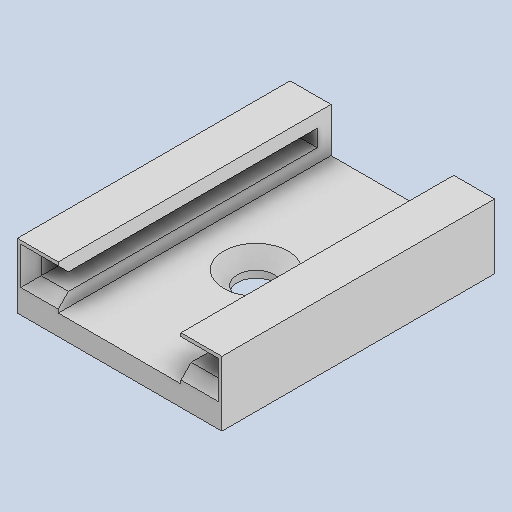
# Autodesk Inventor part: spodok_drazka
Saved by Autodesk Inventor 2025 (Build 290162000, 162)
## iProperties
Created: 2025-09-19
Part Number: spodok_drazka
Material: Generic
Document SubType Name: Modeling
Designer: Pravoslav
Density: 1 g/cm^3
Appearance: Default
Author: Pravoslav
Autodesk Inventor part; units mm, degrees
ref_plane "YZ Plane" through (0, 0, 0) normal (1, 0, 0) x (0, 1, 0)
ref_plane "XZ Plane" through (0, 0, 0) normal (0, 1, 0) x (-1, 0, 0)
ref_plane "XY Plane" through (0, 0, 0) normal (0, 0, 1) x (1, 0, 0)
sketch "Sketch1" plane through (0, 0, 0) normal (0, 1, 0) x (-1, 0, 0)
  line L0 (15, 20) -> (-15, 20)
  line L1 (-15, 20) -> (-15, -20)
  line L2 (-15, -20) -> (15, -20)
  line L3 (15, -20) -> (15, 20)
  line L4 (15, 20) -> (-15, -20) construction
  line L5 (-15, 20) -> (15, -20) construction
  circle A0 centre (0, 0) radius 2.75
  dimension "d0" = 30
  dimension "d1" = 40
  dimension "d2" = 5.5
  constraints: 12 end point, 2 midpoint, 2 parallel, 1 centre point, 1 coincident, 1 horizontal, 1 perpendicular
  measures "d0" distance of L2.end L1.end
  measures "d1" distance of L1.end L0.end
  measures "d2" diameter of A0
extrude "Extrusion1" add sketch "Sketch1" along normal blind 3
chamfer "Chamfer1" distance 2 angle 45 1 edges at (2.75, 3, 0)
sketch "Sketch2" plane through (0, 3, 0) normal (0, 1, 0) x (1, 0, 0)
  line L0 (-15, -20) -> (15, -20) projected
  line L1 (15, 20) -> (-15, 20) projected
  line L2 (-15, -20) -> (-9, -20)
  line L3 (-9, -20) -> (-9, 20)
  line L4 (-9, 20) -> (-15, 20)
  line L5 (-15, 20) -> (-15, -20)
  line L6 (15, -20) -> (15, 20) projected
  line L7 (15, -20) -> (9, -20)
  line L8 (9, -20) -> (9, 20)
  line L9 (9, 20) -> (15, 20)
  line L10 (15, 20) -> (15, -20)
  point P0 (0, 0)
  point P1 (9, 20)
  dimension "d8" = 6
  dimension "d9" = 6
  constraints: 16 end point, 4 parallel, 2 horizontal, 2 perpendicular, 2 point on line
  measures "d8" distance between parallel lines of L5 L3
  measures "d9" distance between parallel lines of L6 L8
extrude "Extrusion2" add sketch "Sketch2" along normal blind 2 contours L5 L1 L3 L0 | L8 L1 L6 L0
sketch "Sketch3" plane through (0, 5, 0) normal (0, 1, 0) x (1, 0, 0)
  line L0 (-15, -20) -> (-9, -20) projected
  line L1 (15, 20) -> (-15, 20) projected
  line L2 (-15, -20) -> (-13, -20)
  line L3 (-13, -20) -> (-13, 20)
  line L4 (-13, 20) -> (-15, 20)
  line L5 (-15, 20) -> (-15, -20)
  line L6 (15, -20) -> (13, -20)
  line L7 (13, -20) -> (13, 20)
  line L8 (13, 20) -> (15, 20)
  line L9 (15, 20) -> (15, -20)
  line L10 (15, -20) -> (15, 20) projected
  line L11 (-9, -20) -> (-9, 20) projected
  line L12 (-15, 20) -> (-9, 20)
  line L13 (-9, 20) -> (-9, 18)
  line L14 (-9, 18) -> (-15, 18)
  line L15 (-15, 18) -> (-15, 20)
  line L16 (9, 20) -> (9, -20) projected
  line L17 (15, 20) -> (9, 20)
  line L18 (9, 20) -> (9, 18)
  line L19 (9, 18) -> (15, 18)
  line L20 (15, 18) -> (15, 20)
  point P0 (0, 0)
  point P1 (13, 18)
  point P2 (-13, 18)
  dimension "d12" = 2
  dimension "d13" = 2
  dimension "d14" = 0
  dimension "d15" = 2
  constraints: 32 end point, 8 parallel, 6 point on line, 4 horizontal, 4 perpendicular
  measures "d12" distance between parallel lines of L5 L3
  measures "d13" distance between parallel lines of L7 L9
  measures "d14" distance between parallel lines of L10 L9
  measures "d15" distance between parallel lines of L1 L14
extrude "Extrusion3" add sketch "Sketch3" along normal blind 2.5 contours L5 L14 L3 L0 | L1 L7 L19 L16 | L5 L1 L3 L14 | L3 L1 L11 L14 | L1 L9 L19 L7 | L19 L9 L6 L7
sketch "Sketch4" plane through (0, 7.5, 0) normal (0, 1, 0) x (1, 0, 0)
  line L0 (-15, 20) -> (-15, -20) projected
  line L1 (15, 20) -> (-15, 20) projected
  line L2 (-15, -20) -> (-9, -20)
  line L3 (-9, -20) -> (-9, 20)
  line L4 (-9, 20) -> (-15, 20)
  line L5 (-15, 20) -> (-15, -20)
  line L6 (15, -20) -> (15, 20) projected
  line L7 (9, -20) -> (9, 20) projected
  line L8 (15, 20) -> (9, 20)
  line L9 (9, 20) -> (9, -20)
  line L10 (9, -20) -> (15, -20)
  line L11 (15, -20) -> (15, 20)
  line L12 (-9, 18) -> (-9, 20) projected
  point P0 (0, 0)
  dimension "d18" = 0
  constraints: 16 end point, 4 parallel, 2 horizontal, 2 perpendicular, 1 point on line
  measures "d18" distance between parallel lines of L12 L3
extrude "Extrusion4" add sketch "Sketch4" along normal blind 2
chamfer "Chamfer2" distance 1.5 angle 45 6 edges at (-13, 6.25, 20) (-11, 7.5, 20) (-11, 5, 20) (11, 5, 20) (13, 6.25, 20) (11, 7.5, 20)
body "Solid1"
